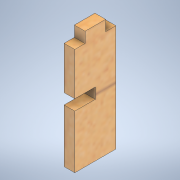
# Autodesk Inventor part: HalterungServoHochSeitlich2
Saved by Autodesk Inventor 2020.3 (Build 243373010, 373A)
## iProperties
Created: 2020-12-10
Part Number: HalterungServoHochSeitlich2
Material: Generisch
Document SubType Name: Modeling
Designer: Stefan
Density: 1 g/cm^3
Appearance: Pappel
Author: Stefan
Autodesk Inventor part; units mm, degrees
ref_plane "YZ Plane" through (0, 0, 0) normal (1, 0, 0) x (0, 1, 0)
ref_plane "XZ Plane" through (0, 0, 0) normal (0, 1, 0) x (-1, 0, 0)
ref_plane "XY Plane" through (0, 0, 0) normal (0, 0, 1) x (1, 0, 0)
sketch "Skizze1" plane through (0, 0, 0) normal (1, 0, 0) x (0, 1, 0)
  line L0 (0, 0) -> (100, 0)
  line L1 (0, 38.5) -> (0, 0)
  line L2 (100, 28.875) -> (110, 28.875)
  line L3 (110, 28.875) -> (110, 9.625)
  line L4 (110, 9.625) -> (100, 9.625)
  line L5 (100, 0) -> (100, 9.625)
  line L6 (100, 28.875) -> (100, 38.5)
  line L7 (60, 38.5) -> (60, 19.25)
  line L8 (60, 19.25) -> (50, 19.25)
  line L9 (50, 19.25) -> (50, 38.5)
  line L10 (100, 38.5) -> (60, 38.5)
  line L11 (50, 38.5) -> (0, 38.5)
  dimension "d0" = 100
  dimension "d1" = 38.5
  dimension "d2" = 10
  dimension "d3" = 19.25
  dimension "d5" = 10
  dimension "d6" = 19.25
  dimension "d7" = 50
  constraints: 24 end point, 6 parallel, 3 perpendicular, 2 horizontal
  measures "d0" distance of L1.start L6.end
  measures "d1" distance of L0.end L6.end
  measures "d2" distance of L3.end L4.end
  measures "d3" distance of L2.end L3.end
  measures "d5" distance of L7.end L8.end
  measures "d6" distance of L7.start L7.end
  measures "d7" distance between parallel lines of L1 L9
extrude "Extrusion1" add sketch "Skizze1" along normal blind 10
